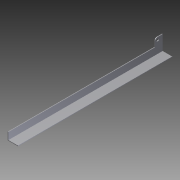
# Autodesk Inventor part: 8 ball top roller L frame
Saved by Autodesk Inventor 2012 (Build 160160000, 160)
## iProperties
Created: 2013-10-29
Part Number: 8 ball top roller L frame
Material: Default
Document SubType Name: Modeling
Designer: Bryce
Density: 1 g/cm^3
Author: Bryce
Autodesk Inventor part; units mm, degrees
ref_plane "YZ Plane" through (0, 0, 0) normal (1, 0, 0) x (0, 1, 0)
ref_plane "XZ Plane" through (0, 0, 0) normal (0, 1, 0) x (-1, 0, 0)
ref_plane "XY Plane" through (0, 0, 0) normal (0, 0, 1) x (1, 0, 0)
sketch "Sketch1" plane through (0, 0, 0) normal (0, 0, 1) x (1, 0, 0)
  line L0 (0, 0) -> (25.4, 0)
  line L1 (25.4, 0) -> (25.4, 1.5875)
  line L2 (1.5875, 38.1) -> (0, 38.1)
  line L3 (0, 38.1) -> (0, 0)
  line L4 (1.5875, 38.1) -> (1.5875, 1.5875)
  line L5 (1.5875, 1.5875) -> (25.4, 1.5875)
  dimension "d0" = 1.5875
  dimension "d1" = 1.5875
  dimension "d2" = 25.4
  dimension "d3" = 38.1
  constraints: 12 end point, 2 parallel, 1 horizontal, 1 perpendicular
  measures "d0" distance between parallel lines of L4 L3
  measures "d1" distance between parallel lines of L0 L5
  measures "d2" distance of L0.start L0.end
  measures "d3" distance of L2.end L0.start
extrude "Extrusion1" add sketch "Sketch1" along normal blind 384.175
sketch "Sketch2" plane through (0, 0, 0) normal (-1, 0, 0) x (0, 0, 1)
  line L0 (384.175, 0) -> (384.175, 38.1) projected
  line L1 (0, 38.1) -> (384.175, 38.1) projected
  line L2 (0, 38.1) -> (0, 0) projected
  line L3 (0, 0) -> (384.175, 0) projected
  line L4 (19.05, 38.1) -> (19.05, 19.05)
  line L5 (19.05, 19.05) -> (384.175, 19.05)
  circle A0 centre (12.7, 31.75) radius 3.175
  arc A1 (19.05, 31.75) -> (12.7, 38.1) centre (12.7, 31.75) ccw
  dimension "d6" = 19.05
  dimension "d7" = 19.05
  dimension "d8" = 6.35
  dimension "d9" = 12.7
  dimension "d10" = 6.35
  constraints: 4 end point, 3 point on line, 2 centre point, 2 perpendicular, 2 point on circle, 1 coincident, 1 midpoint, 1 tangent
  measures "d6" distance between parallel lines of L4 L2
  measures "d7" distance of L4.start L4.end
  measures "d8" diameter of A0
  measures "d9" distance from line of L2 A0.centre
  measures "d10" distance from line of L1 A0.centre
extrude "Extrusion2" cut sketch "Sketch2" against normal blind 25.4 contours L5 L4 L1 L0 | L4 A1 L1 | A0
equation "\"d0\" = d1"
body "Solid1"
